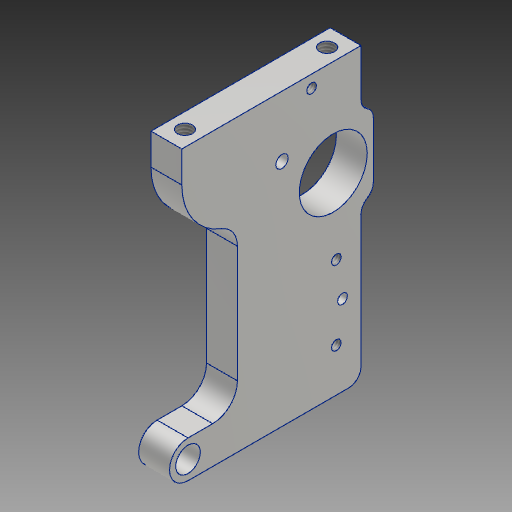
# Autodesk Inventor part: Dribbler Seite
Saved by Autodesk Inventor 2019.4 (Build 234330000, 330)
## iProperties
Part Number: Dribbler Seite
Material: Aluminium 6061
Document SubType Name: Modeling
Designer: rYan
Density: 2.7 g/cm^3
Appearance: Aluminium - flach
Mass: 13.678 g
Surface Area: 33.5514 cm^2
Volume: 5.06591 cm^3
Author: rYan
Autodesk Inventor part; units mm, degrees
ref_plane "YZ Plane" through (0, 0, 0) normal (1, 0, 0) x (0, 1, 0)
ref_plane "XZ Plane" through (0, 0, 0) normal (0, 1, 0) x (-1, 0, 0)
ref_plane "XY Plane" through (0, 0, 0) normal (0, 0, 1) x (1, 0, 0)
sketch "Skizze1" plane through (0, 0, 0) normal (1, 0, 0) x (0, 1, 0)
  circle A0 centre (-22.8, 48.5) radius 11 construction
  circle A1 centre (-4.5, 41.3809) radius 6.5 construction
  line L0 (-97.6965, 0) -> (58.2827, 0) projected
  circle A2 centre (14.5, 21.5) radius 21.5 construction
  line L1 (-28, 10) -> (0, 10)
  line L2 (0, 10) -> (0, 35.3809)
  line L3 (-7, 0) -> (-7, 21.5) construction
  circle A3 centre (-4.5, 41.3809) radius 6 construction
  circle A4 centre (-4.5, 41.3809) radius 5 construction
  line L4 (-56.6136, 29) -> (0, 29) construction
  arc A5 (-28, 16) -> (-28, 10) centre (-28, 13) ccw
  line L5 (-75.4137, 30) -> (0, 30) construction
  line L6 (-28, 16) -> (-20, 16)
  line L7 (-20, 16) -> (-20, 42)
  line L8 (-20, 42) -> (-29, 42)
  line L9 (-29, 42) -> (-29, 57)
  circle A6 centre (-28, 13) radius 2
  circle A7 centre (-4.5, 41.3809) radius 5.5
  circle A8 centre (-22.8, 48.5) radius 0.5
  circle A9 centre (-3, 23) radius 0.8
  line L10 (14.5, 21.5) -> (-7, 21.5) construction
  line L11 (-29, 57) -> (0, 57)
  line L12 (-4.5, 41.3809) -> (-28, 13) construction
  line L13 (14.5, 21.5) -> (14.5, 20.5) construction
  line L14 (14.5, 20.5) -> (-4.5, 41.3809) construction
  circle A10 centre (-22.8, 48.5) radius 5 construction
  circle A11 centre (-12.7907, 47.1492) radius 5.1 construction
  circle A12 centre (-12.7907, 47.1492) radius 5.6 construction
  circle A13 centre (-12.7907, 47.1492) radius 1
  line L15 (0, 35.3809) -> (2, 35.3809)
  line L16 (2, 35.3809) -> (2, 47.3809)
  line L17 (2, 47.3809) -> (0, 47.3809)
  line L18 (0, 47.3809) -> (0, 57)
  line L19 (1, 41.3809) -> (-10, 41.3809) construction
  point P0 (0, 0)
  dimension "d4" = 43
  dimension "d0" = 22
  dimension "d2" = 13
  dimension "d5" = 10
  dimension "d6" = 7
  dimension "d7" = 12
  dimension "d8" = 10
  dimension "d9" = 29
  dimension "d11" = 30
  dimension "d12" = 4
  dimension "d14" = 6
  dimension "d15" = 28
  dimension "d16" = 20
  dimension "d17" = 42
  dimension "d19" = 29
  dimension "d20" = 11
  dimension "d33" = 1
  dimension "d34" = 48.5
  dimension "d36" = 1.6
  dimension "d37" = 3
  dimension "d54" = 57
  dimension "d58" = 1
  dimension "d59" = 81.925
  dimension "d65" = 10
  dimension "d66" = 10.2
  dimension "d67" = 0.5
  dimension "d68" = 2
  dimension "d69" = 2
  dimension "d70" = 6
  dimension "d72" = 1.5
  dimension "d73" = 22.8
  constraints: 38 end point, 13 centre point, 8 coincident, 8 horizontal, 7 perpendicular, 5 tangent, 4 point on circle, 4 point on line, 4 vertical, 1 collinear, 1 horizontal alignment, 1 midpoint, 4 other
  measures "d0" diameter of A0
  measures "d2" diameter of A1
  measures "d5" distance between parallel lines of L1 L0
  measures "d6" distance between parallel lines of L2 L3
  measures "d7" diameter of A3
  measures "d8" diameter of A4
  measures "d9" distance between parallel lines of L0 L4
  measures "d11" distance between parallel lines of L0 L5
  measures "d12" diameter of A6
  measures "d14" diameter of A5
  measures "d15" distance from line of A5.centre L2
  measures "d16" distance between parallel lines of L2 L7
  measures "d17" distance between parallel lines of L0 L8
  measures "d19" distance between parallel lines of L2 L9
  measures "d20" diameter of A7
  measures "d33" diameter of A8
  measures "d34" distance from line of L0 A0.centre
  measures "d36" diameter of A9
  measures "d37" distance from line of L2 A9.centre
  measures "d54" distance between parallel lines of L0 L11
  measures "d58" distance of L10.start L13.end
  measures "d59" angle of L12 L14
  measures "d65" diameter of A10
  measures "d66" diameter of A11
  measures "d67" radial gap between concentric circles of A12 A11
  measures "d68" diameter of A13
  measures "d69" distance of L16.end L17.end
  measures "d70" distance between parallel lines of L17 L19
  measures "d72" distance from line of A9.centre L10
  measures "d73" distance from line of A0.centre L18
extrude "Extrusion1" add sketch "Skizze1" along normal mid plane 5 contours A5 L6 L7 L8 L9 L11 L18 L17 L16 L15 L2 L1 | A8
sketch "Skizze2" plane through (-2.5, -29, 57) normal (0, 0, 1) x (1, 0, 0)
  line L0 (0, 0) -> (5, 0) projected
  line L1 (5, 5) -> (5, 0) projected
  line L2 (0, 0) -> (0, 5) projected
  line L3 (2.5, 29) -> (2.5, 0) construction
  line L4 (0, 0) -> (5, 0) construction
  line L5 (0, 5) -> (5, 5) projected
  line L6 (0, 29) -> (5, 29) projected
  line L7 (0, 29) -> (5, 29) projected
  point P0 (2.5, 26)
  point P1 (2.5, 3)
  dimension "d25" = 23
  dimension "d74" = 3
  constraints: 2 end point, 2 point on line, 1 midpoint
  measures "d25" distance of point (2.5, 3) point (2.5, 26)
  measures "d74" distance from line of L6 point (2.5, 26)
hole "Bohrung1" at (0, -3, 57) at (0, -26, 57) direction (0, 0, -1) diameter 2.459 depth 7 tip angle 118 thread size "M3x0.5" class "6H" standard "ISO Metric profile"
fillet "Rundung1" radius 10 1 edges at (0, -29, 42)
sketch "Skizze3" plane through (-2.5, 0, 0) normal (-1, 0, 0) x (0, 0, 1)
  circle A0 centre (23, -3) radius 0.8 projected
  line L0 (29, -4) -> (17, -4) construction
  circle A1 centre (23, -3) radius 0.8 construction
  line L1 (23, -4) -> (23, -3) construction
  point P0 (0, 0)
  point P1 (55, -8)
  dimension "d38" = 12
  dimension "d39" = 1
  dimension "d40" = 32
  dimension "d41" = 5
  constraints: 4 end point, 2 coincident, 1 horizontal, 1 midpoint, 1 vertical
  measures "d38" distance of L0.start L0.end
  measures "d39" distance from line of L0 A0.centre
  measures "d40" horizontal distance of point (55, -8) A0.centre
  measures "d41" vertical distance of point (55, -8) A0.centre
hole "Bohrung2" at (-2.5, -4, 17) at (-2.5, -4, 29) at (-2.5, -8, 55) direction (1, 0, 0) diameter 1.567 end through all thread size "M2x0.4" class "6H" standard "ISO Metric profile"
fillet "Rundung2" radius 4 2 edges at (0, -20, 42) (0, -20, 16)
fillet "Rundung3" radius 2 1 edges at (0, 0, 10)
fillet "Rundung4" radius 2 4 edges at (0, 0, 47.3809) (0, 2, 47.3809) (0, 2, 35.3809) (0, 0, 35.3809)
